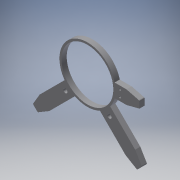
# Autodesk Inventor part: CircularHeadbar_large_simple
Saved by Autodesk Inventor 2016 (Build 200138000, 138)
## iProperties
Created: 2015-02-26
Part Number: CircularHeadbar_large_simple
Material: Generic
Document SubType Name: Modeling
Designer: ChurchlandLab
Density: 1 g/cm^3
Sheet Metal Rule: Default
Appearance: Default
Author: ChurchlandLab
Autodesk Inventor part; units mm, degrees
ref_plane "YZ Plane" through (0, 0, 0) normal (1, 0, 0) x (0, 1, 0)
ref_plane "XZ Plane" through (0, 0, 0) normal (0, 1, 0) x (-1, 0, 0)
ref_plane "XY Plane" through (0, 0, 0) normal (0, 0, 1) x (1, 0, 0)
sketch "Sketch1" plane through (0, 0, 0) normal (0, 0, 1) x (1, 0, 0)
  line L0 (-0.0012, 9.6891) -> (-0.0012, -0.0155) construction
  circle A0 centre (-0.0012, -0.0155) radius 6.35
  line L1 (9.3601, -12.4316) -> (3.0739, -6.1454)
  line L2 (5.5879, -3.9897) -> (11.6952, -10.0969)
  line L3 (9.3601, -12.4316) -> (12.1799, -14.1019)
  line L4 (12.1799, -14.1019) -> (13.3653, -12.9165)
  line L5 (13.3653, -12.9165) -> (11.6952, -10.0969)
  line L6 (13.4673, -0.0155) -> (-6.3512, -0.0155) construction
  arc A1 (-3.0764, -6.1454) -> (3.0739, -6.1454) centre (-0.0012, -0.0155) ccw
  arc A2 (0.9828, -6.8026) -> (3.0739, -6.1454) centre (-0.0012, -0.0155) ccw
  arc A3 (-0.0012, 6.8425) -> (-5.5904, -3.9897) centre (-0.0012, -0.0155) ccw
  arc A4 (-6.8132, -0.8093) -> (-5.5904, -3.9897) centre (-0.0012, -0.0155) ccw
  arc A5 (5.5879, -3.9897) -> (6.6536, -1.6723) centre (-0.0012, -0.0155) ccw
  arc A6 (6.6536, 1.6412) -> (3.738, 5.7334) centre (-0.0012, -0.0155) ccw
  arc A7 (5.5879, -3.9897) -> (6.6536, -1.6723) centre (-0.0012, -0.0155) ccw
  arc A8 (6.6536, 1.6412) -> (-0.0012, 6.8425) centre (-0.0012, -0.0155) ccw
  line L7 (5.5879, -3.9897) -> (21.5848, -3.9897) construction
  line L8 (-9.3626, -12.4316) -> (-3.0764, -6.1454)
  line L9 (-5.5904, -3.9897) -> (-11.6977, -10.0969)
  line L10 (-9.3626, -12.4316) -> (-12.1824, -14.1019)
  line L11 (-12.1824, -14.1019) -> (-13.3678, -12.9165)
  line L12 (-13.3678, -12.9165) -> (-11.6977, -10.0969)
  line L13 (9.5746, 1.6412) -> (12.7483, 0.8287)
  line L14 (6.6536, 1.6412) -> (9.5746, 1.6412)
  line L15 (9.5746, -1.6723) -> (12.7483, -0.8598)
  line L16 (6.6536, -1.6723) -> (9.5746, -1.6723)
  circle A9 centre (7.9363, -0.8093) radius 0.254
  circle A10 centre (7.9363, 0.7782) radius 0.254
  circle A11 centre (-5.4113, -6.1454) radius 0.508
  line L17 (12.7483, 0.8287) -> (12.7483, -0.8598)
  circle A12 centre (5.4088, -6.1454) radius 0.508
  point P0 (13.4229, -0.6871)
  point P1 (13.4673, -0.0008)
  dimension "d35" = 12.7
  dimension "d72" = 8.89
  dimension "d73" = 3.2774
  dimension "d77" = 194.36
  dimension "d78" = 1.6764
  dimension "d115" = 90
  dimension "d128" = 165.64
  dimension "d148" = 0.508
  dimension "d154" = 3.302
  dimension "d160" = 3.276
  dimension "d166" = 0.508
  dimension "d168" = 7.9375
  dimension "d169" = 0.863
  dimension "d176" = 1.016
  dimension "d182" = 3.3135
  dimension "d184" = 1.6885
  dimension "d191" = 2.921
  dimension "d234" = 24.3623
  constraints: 36 end point, 16 point on circle, 12 centre point, 11 symmetric about line, 3 point on line, 2 perpendicular, 1 coincident, 1 horizontal, 1 horizontal alignment, 1 vertical, 4 other
  measures "d72" distance of L1.end L1.start
  measures "d73" distance of L1.start L3.end
  measures "d78" distance of L3.end L4.end
  measures "d115" angle of L0 L6
  measures "d128" angle of L5 L2
  measures "d154" distance between parallel lines of L1 L2
  measures "d160" distance of L13.start L13.end
  measures "d166" diameter of A9
  measures "d168" horizontal distance of L0.end A9.centre
  measures "d169" distance from line of L16 A9.centre
  measures "d176" diameter of A11
  measures "d182" distance of L16.start L14.start
  measures "d184" distance of L13.end L15.end
  measures "d191" distance of L14.start L13.start
  measures "d234" distance of L10.end L3.end
extrude "Extrusion8" add sketch "Sketch1" along normal blind 1.27
fillet "Fillet57" radius 0.254 1 edges at (-12.1824, -14.1019, 0.635)
fillet "Fillet58" radius 0.254 1 edges at (-13.3678, -12.9165, 0.635)
fillet "Fillet59" radius 0.254 1 edges at (13.3653, -12.9165, 0.635)
fillet "Fillet60" radius 0.254 1 edges at (12.1799, -14.1019, 0.635)
fillet "Fillet63" radius 0.254 1 edges at (12.7483, 0.8287, 0.635)
equation "\"BendRadius\" = Thickness"
equation "\"BendReliefWidth\" = Thickness"
equation "\"BendReliefDepth\" = 0.5 * Thickness"
equation "\"CornerReliefSize\" = 4 * Thickness"
equation "\"MinimumRemnant\" = 2 * Thickness"
equation "\"TransitionRadius\" = BendRadius"
equation "\"JacobiRadiusSize\" = BendRadius"
equation "\"GapSize\" = Thickness"
equation "\"Thickness\" = 3.048"
body "Solid7"
